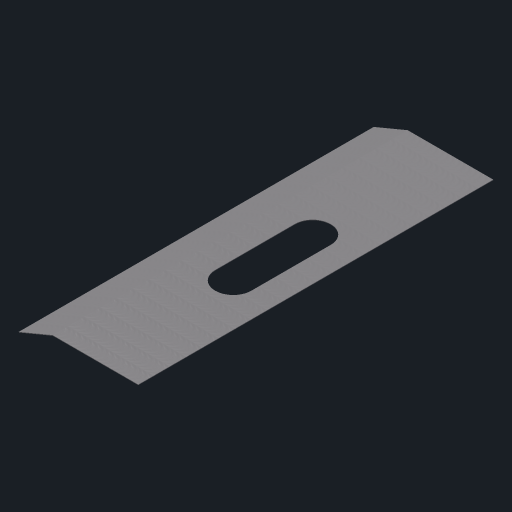
# Autodesk Inventor part: CHAPA_1
Saved by Autodesk Inventor 2024.3 (Build 283343000, 343)
## iProperties
Created: 2024-06-14
Part Number: CHAPA_1
Material: Steel, Mild, Welded
Document SubType Name: Sheet Metal
Designer: Niler
Density: 7.85 g/cm^3
Sheet Metal Rule: Default_mm
Appearance: Weld - Steel Mild
Flat Pattern Width: 33.8653 cm
Flat Pattern Length: 98.3 cm
Flat Pattern Area: 3328.96 cm^2
Sheet Metal Width: 338.653 mm
Sheet Metal Length: 983.000 mm
Sheet Metal Area: 332895.650 mm^2
Author: Niler
Autodesk Inventor part; units mm, degrees
ref_plane "YZ Plane" through (0, 0, 0) normal (1, 0, 0) x (0, 1, 0)
ref_plane "XZ Plane" through (0, 0, 0) normal (0, 1, 0) x (-1, 0, 0)
ref_plane "XY Plane" through (0, 0, 0) normal (0, 0, 1) x (1, 0, 0)
sketch "Sketch1" plane through (0, 0, 0) normal (0, 1, 0) x (-1, 0, 0)
  line L0 (-118.5, 491.5) -> (118.5, 491.5)
  line L1 (118.5, 491.5) -> (118.5, -491.5)
  line L2 (118.5, -491.5) -> (-118.5, -491.5)
  line L3 (-118.5, -491.5) -> (-118.5, 491.5)
  line L4 (-118.5, 491.5) -> (118.5, -491.5) construction
  line L5 (118.5, 491.5) -> (-118.5, -491.5) construction
  point P0 (0, 0)
  dimension "d0" = 983
  dimension "d1" = 237
extrude "Plate1" add sketch "Sketch1" along normal blind 1.5
sketch "Sketch2" plane through (0, 1.5, 0) normal (0, 1, 0) x (1, 0, 0)
  line L0 (0, -110) -> (0, 110) construction
  line L1 (50, -110) -> (50, 110)
  line L2 (-50, 110) -> (-50, -110)
  arc A0 (-50, -110) -> (50, -110) centre (0, -110) ccw
  arc A1 (50, 110) -> (-50, 110) centre (0, 110) ccw
  point P0 (0, 0)
  dimension "d3" = 50
  dimension "d4" = 220
  constraints: 8 end point, 4 point on circle, 4 tangent, 2 centre point, 1 midpoint, 1 parallel, 1 vertical
  measures "d3" radius of A0
  measures "d4" distance of L0.end L0.start
extrude "Extrusion1" cut sketch "Sketch2" against normal through all
sketch "Sketch3" plane through (-117.9231, 0.1154, -491.5) normal (-0.3846176, 0.923076, 0) x (-0.923076, -0.3846176, 0)
  line L0 (0, 983) -> (0, 0)
  line L1 (0, 0) -> (102, 0)
  line L2 (102, 0) -> (102, 983)
  line L3 (102, 983) -> (0, 983)
  constraints: 6 end point, 1 horizontal, 1 perpendicular, 1 vertical
edge flange "Flange1" height 102 angle 22.62 thickness 1.5 bend radius 1.5 thickness toward (-0.3846176, 0.923076, 0) relief straight relief width 1.5 relief depth 0.75 edges at (-118.5, 0, 0) wall of the first edge with corners at (-117.9231, 0.1154, 491.5) (-117.9231, 0.1154, -491.5) (-212.0768, -39.1156, -491.5) (-212.0768, -39.1156, 491.5)
bend "Bend1"
corner "Corner1"
equation "\"d2\" = Thickness"
equation "\"d7\" = BendReliefWidth"
equation "\"d8\" = BendReliefDepth"
equation "\"d9\" = MinimumRemnant"
equation "\"d10\" = TransitionRadius"
equation "\"d13\" = BendRadius"
equation "\"d14\" = CornerReliefSize"
equation "\"d15\" = GapSize"
equation "\"d16\" = JacobiRadiusSize"
equation "\"BendRadius\" = Thickness"
equation "\"BendReliefWidth\" = Thickness"
equation "\"BendReliefDepth\" = 0.5 * Thickness"
equation "\"CornerReliefSize\" = 4 * Thickness"
equation "\"MinimumRemnant\" = 2 * Thickness"
equation "\"TransitionRadius\" = BendRadius"
equation "\"JacobiRadiusSize\" = BendRadius"
equation "\"GapSize\" = Thickness"
equation "\"Thickness\" = 1.5"
body "Solid1"
